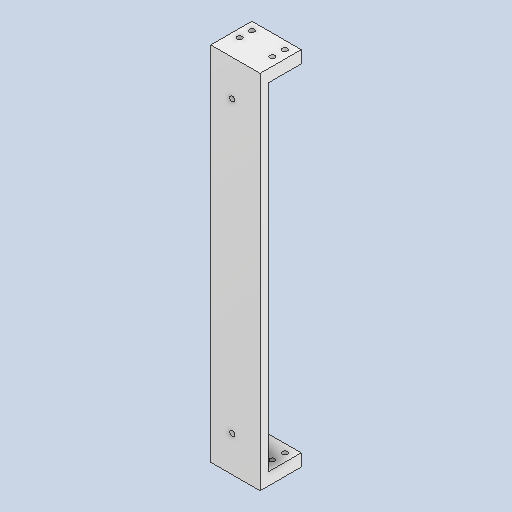
# Autodesk Inventor part: Back_Cover
Saved by Autodesk Inventor 2024.3 (Build 283343000, 343)
## iProperties
Created: 2024-09-08
Part Number: Back_Cover
Material: LCP 플라스틱
Document SubType Name: Modeling
Designer: ASUS
Density: 1.626 g/cm^3
Appearance: 매끄러움 - 흰색
Mass: 34.5185 g
Surface Area: 123.096 cm^2
Volume: 21.2291 cm^3
Author: ASUS
Autodesk Inventor part; units mm, degrees
ref_plane "YZ Plane" through (0, 0, 0) normal (1, 0, 0) x (0, 1, 0)
ref_plane "XZ Plane" through (0, 0, 0) normal (0, 1, 0) x (-1, 0, 0)
ref_plane "XY Plane" through (0, 0, 0) normal (0, 0, 1) x (1, 0, 0)
sketch "스케치1" plane through (0, 0, 0) normal (0, 0, 1) x (1, 0, 0)
  line L0 (-12, 88) -> (12, 88)
  line L1 (12, 88) -> (12, -88)
  line L2 (12, -88) -> (-12, -88)
  line L3 (-12, -88) -> (-12, 88)
  line L4 (-12, 88) -> (12, -88) construction
  line L5 (12, 88) -> (-12, -88) construction
  point P0 (0, 0)
  dimension "d0" = 24
  dimension "d1" = 176
  constraints: 12 end point, 2 midpoint, 2 parallel, 1 horizontal, 1 perpendicular
  measures "d0" distance of L1.end L2.end
  measures "d1" distance of L0.end L1.end
extrude "돌출1" add sketch "스케치1" along normal blind 4
sketch "스케치2" plane through (12, -88, 0) normal (1, 0, 0) x (0, 0, -1)
  line L0 (0, 0) -> (0, 176) projected
  line L1 (0, 176) -> (-4, 176) projected
  line L2 (-4, 0) -> (-4, 176) projected
  line L3 (0, 0) -> (-4, 0) projected
  line L4 (-4, 0) -> (-4, 176) projected
  line L5 (-4, 176) -> (16, 176)
  line L6 (16, 176) -> (16, 170)
  line L7 (16, 170) -> (-4, 170)
  line L8 (-4, 170) -> (-4, 176)
  line L9 (-4, 0) -> (16, 0)
  line L10 (16, 0) -> (16, 6)
  line L11 (16, 6) -> (-4, 6)
  line L12 (-4, 6) -> (-4, 0)
  point P0 (0, 88)
  point P1 (0, 6)
  point P2 (0, 170)
  dimension "d4" = 20
  dimension "d5" = 6
  dimension "d6" = 20
  dimension "d7" = 6
  constraints: 16 end point, 4 parallel, 2 horizontal, 2 perpendicular
  measures "d4" distance of L6.end L7.end
  measures "d5" distance of L5.end L6.end
  measures "d6" distance of L11.end L10.end
  measures "d7" distance of L10.end L9.end
extrude "돌출2" add sketch "스케치2" against normal up to surface (24 mm away) contours L0 L11 L10 L9 | L0 L5 L6 L7
sketch "스케치3" plane through (-12, -88, 4) normal (0, -1, 0) x (1, 0, 0)
  line L0 (24, -20) -> (24, 0) projected
  line L1 (0, 0) -> (24, 0) projected
  line L2 (0, 0) -> (0, -20) projected
  line L3 (24, -20) -> (0, -20) projected
  line L4 (4, -16) -> (4, -4)
  line L5 (4, -4) -> (20, -4)
  line L6 (20, -4) -> (20, -16)
  line L7 (20, -16) -> (4, -16)
  circle A0 centre (20, -16) radius 1.25
  circle A1 centre (4, -16) radius 1.25
  circle A2 centre (20, -4) radius 1.25
  circle A3 centre (4, -4) radius 1.25
  circle A4 centre (20, -10) radius 1.25
  circle A5 centre (4, -10) radius 1.25
  point P0 (12, -4)
  dimension "d10" = 4
  dimension "d11" = 2.5
  dimension "d12" = 2.5
  dimension "d13" = 2.5
  dimension "d14" = 2.5
  dimension "d15" = 2.5
  dimension "d16" = 2.5
  constraints: 8 end point, 6 centre point, 4 coincident, 2 midpoint, 3 other
  measures "d10" distance between parallel lines of L3 L7
  measures "d11" diameter of A0
  measures "d12" diameter of A1
  measures "d13" diameter of A2
  measures "d14" diameter of A3
  measures "d15" diameter of A4
  measures "d16" diameter of A5
extrude "돌출3" cut sketch "스케치3" against normal through all contours L7 A1 L4 | L4 A1 L7 | A5 L4 | L4 A5 | A0 L6 L7 | L7 L6 A0 | A4 L6 | L6 A4
sketch "스케치6" plane through (0, 0, 4) normal (0, 0, 1) x (1, 0, 0)
  circle A0 centre (-1.5, -70.5) radius 1.25 projected
  line L0 (6, -62) -> (6, -79) projected
  line L1 (-9.5, -79) -> (6, -79) projected
  line L2 (-9.5, -79) -> (-9.5, -62) projected
  line L3 (6, -62) -> (-9.5, -62) projected
  circle A1 centre (-1.5, 70.5) radius 1.25 projected
  line L4 (6, 62) -> (6, 79) projected
  line L5 (6, 62) -> (-9.5, 62) projected
  line L6 (-9.5, 79) -> (-9.5, 62) projected
  line L7 (-9.5, 79) -> (6, 79) projected
  point P0 (0, 0)
extrude "돌출6" cut sketch "스케치6" against normal blind 10 contours A0 | A1
